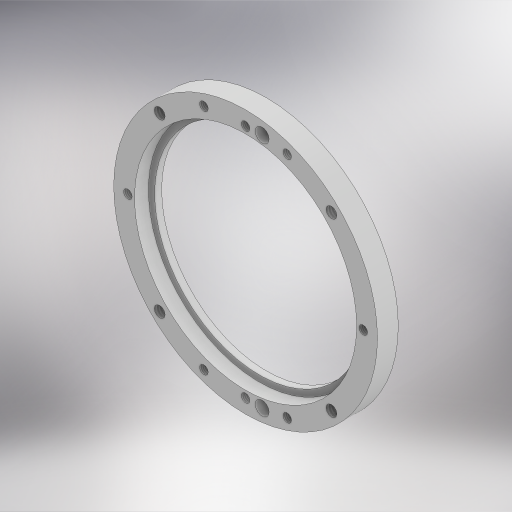
# Autodesk Inventor part: LS-001
Saved by Autodesk Inventor 2023.4 (Build 274418000, 418)
## iProperties
Created: 2025-03-08
Part Number: LS-001
Material: Generic
Document SubType Name: Modeling
Designer: jmcintyr
Density: 1 g/cm^3
Appearance: Default
Author: jmcintyr
Autodesk Inventor part; units mm, degrees
ref_plane "YZ Plane" through (0, 0, 0) normal (1, 0, 0) x (0, 1, 0)
ref_plane "XZ Plane" through (0, 0, 0) normal (0, 1, 0) x (-1, 0, 0)
ref_plane "XY Plane" through (0, 0, 0) normal (0, 0, 1) x (1, 0, 0)
sketch "Sketch1" plane through (0, 0, 0) normal (0, 0, 1) x (1, 0, 0)
  circle A0 centre (0, 0) radius 60.325
  circle A1 centre (0, 0) radius 47.625
  dimension "d0" = 120.65
  dimension "d1" = 12.7
  constraints: 2 centre point, 1 coincident
  measures "d0" diameter of A0
  measures "d1" radial gap between concentric circles of A0 A1
extrude "Extrusion1" add sketch "Sketch1" against normal blind 9.525
sketch "Sketch2" plane through (0, 0, 0) normal (0, 0, 1) x (1, 0, 0)
  circle A0 centre (0, 0) radius 50.8
  circle A1 centre (0, 0) radius 47.625 projected
  dimension "d4" = 101.6
  constraints: 1 centre point, 1 coincident
  measures "d4" diameter of A0
extrude "Extrusion2" cut sketch "Sketch2" against normal blind 6.35 contours A0 | A1
sketch "Sketch3" plane through (0, 0, 0) normal (0, 0, 1) x (1, 0, 0)
  circle A0 centre (0, 0) radius 53.848 construction
  circle A1 centre (0, 0) radius 60.325 projected
  point P0 (0, 53.848)
  point P1 (-53.848, 0)
  point P2 (0, -53.848)
  point P3 (53.848, 0)
  dimension "d7" = 53.848
  dimension "d10" = 360
  constraints: 1 vertical alignment, 8 other
  measures "d7" distance of point (0, 53.848) point (0, 0)
hole "Hole1" at (0, 53.848, 0) at (-53.848, 0, 0) at (0, -53.848, 0) at (53.848, 0, 0) direction (0, 0, -1) diameter 3.9624 end through all thread size "10-32 UNF" class "2B" standard "ANSI Unified Screw Threads"
sketch "Sketch4" plane through (0, 0, -9.525) normal (0, 0, -1) x (-1, 0, 0)
  circle A0 centre (0, 0) radius 47.9425
  circle A1 centre (0, 0) radius 47.625 projected
  dimension "d19" = 95.885
  constraints: 1 centre point, 1 coincident
  measures "d19" diameter of A0
extrude "Extrusion3" cut sketch "Sketch4" against normal blind 6.35
sketch "Sketch5" plane through (0, 0, 0) normal (0, 0, 1) x (1, 0, 0)
  circle A0 centre (0, 0) radius 55.5625 construction
  line L0 (0, 0) -> (0, 55.5625) construction
  circle A1 centre (0, 0) radius 60.325 construction
  line L1 (-60.325, 0) -> (60.325, 0) construction
  line L2 (-19.05, -52.1947) -> (-19.05, 52.1947) construction
  line L3 (19.05, -52.1947) -> (19.05, 52.1947) construction
  dimension "d22" = 111.125
  dimension "d25" = 19.05
  dimension "d26" = 19.05
  dimension "d47" = 104.394
  constraints: 8 end point, 7 point on circle, 3 coincident, 2 parallel, 1 centre point, 1 horizontal, 1 vertical
  measures "d22" diameter of A0
  measures "d25" distance between parallel lines of L0 L2
  measures "d26" distance between parallel lines of L0 L3
hole "Hole2" at (-19.05, 52.1947, 0) at (19.05, 52.1947, 0) at (-19.05, -52.1947, 0) at (19.05, -52.1947, 0) direction (0, 0, -1) diameter 3.9624 end through all thread size "10-32 UNF" class "2B" standard "ANSI Unified Screw Threads"
sketch "Sketch6" plane through (0, 0, 0) normal (0, 0, 1) x (1, 0, 0)
  circle A0 centre (0, 0) radius 55.5625 construction
  line L0 (0, 0) -> (-39.2886, 39.2886) construction
  line L1 (0, 0) -> (-60.7712, 0) construction
  point P0 (-39.2886, -39.2886)
  point P1 (39.2886, -39.2886)
  point P2 (39.2886, 39.2886)
  dimension "d34" = 111.125
  dimension "d35" = 45
  dimension "d38" = 360
  constraints: 4 end point, 2 coincident, 1 horizontal, 8 other
  measures "d35" angle of L1 L0
hole "Hole3" at (-39.2886, 39.2886, 0) at (-39.2886, -39.2886, 0) at (39.2886, -39.2886, 0) at (39.2886, 39.2886, 0) direction (0, 0, -1) diameter 4.9784 end through all thread size "1/4-20 UNC" class "2B" standard "ANSI Unified Screw Threads"
sketch "Sketch7" plane through (0, 0, 0) normal (0, 0, 1) x (1, 0, 0)
  circle A0 centre (0, 0) radius 54.61 construction
  line L0 (0, 0) -> (0, 54.61) construction
  line L1 (0, 0) -> (7.6002, 54.0785) construction
  circle A1 centre (0, 0) radius 60.325 construction
  line L2 (-60.325, 0) -> (60.325, 0) construction
  circle A2 centre (39.2886, -39.2886) radius 2.4892 projected
  circle A3 centre (-39.2886, 39.2886) radius 2.4892 projected
  circle A4 centre (-39.2886, -39.2886) radius 2.4892 projected
  circle A5 centre (39.2886, 39.2886) radius 2.4892 projected
  circle A6 centre (-19.05, -52.1947) radius 1.9812 projected
  circle A7 centre (-19.05, 52.1947) radius 1.9812 projected
  circle A8 centre (19.05, 52.1947) radius 1.9812 projected
  circle A9 centre (19.05, -52.1947) radius 1.9812 projected
  circle A10 centre (0, -53.848) radius 1.9812 projected
  circle A11 centre (0, 53.848) radius 1.9812 projected
  circle A12 centre (-53.848, 0) radius 1.9812 projected
  circle A13 centre (53.848, 0) radius 1.9812 projected
  circle A14 centre (0, 0) radius 50.8 projected
  circle A15 centre (0, 0) radius 60.325 projected
  point P0 (7.6002, -54.0785)
  dimension "d49" = 109.22
  dimension "d50" = 8
  constraints: 6 end point, 4 point on circle, 2 coincident, 1 centre point, 1 horizontal, 1 symmetric about line
  measures "d49" diameter of A0
  measures "d50" angle of L1 L0
hole "Hole4" at (7.6002, 54.0785, 0) at (7.6002, -54.0785, 0) direction (0, 0, -1) diameter 6.35 end through all
body "Solid1"
